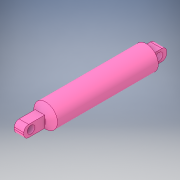
# Autodesk Inventor part: MockShock2
Saved by Autodesk Inventor 2018.2 (Build 222227000, 227)
## iProperties
Created: 2018-03-24
Part Number: MockShock2
Material: Generic
Document SubType Name: Modeling
Designer: MIABo
Density: 1 g/cm^3
Appearance: Default
Author: MIABo
Autodesk Inventor part; units mm, degrees
ref_plane "YZ Plane" through (0, 0, 0) normal (1, 0, 0) x (0, 1, 0)
ref_plane "XZ Plane" through (0, 0, 0) normal (0, 1, 0) x (-1, 0, 0)
ref_plane "XY Plane" through (0, 0, 0) normal (0, 0, 1) x (1, 0, 0)
sketch "Sketch1" plane through (0, 0, 0) normal (0, 0, 1) x (1, 0, 0)
  circle A0 centre (0, 0) radius 7.874
  dimension "d0" = 15.748
  constraints: 1 centre point, 1 coincident
  measures "d0" diameter of A0
extrude "Extrusion1" add sketch "Sketch1" along normal blind 67.31
ref_plane "Work Plane1" through (0, 0, 71.12) normal (0, 0, 1) x (1, 0, 0)
sketch "Sketch3" plane through (0, 0, 71.12) normal (0, 0, 1) x (1, 0, 0)
  circle A0 centre (0, 0) radius 3.81
  dimension "d4" = 7.62
  constraints: 1 centre point, 1 coincident
  measures "d4" diameter of A0
loft "Loft1" add profiles "Sketch3" section 1 edges at (-7.874, 0, 67.31)
ref_plane "Work Plane5" through (0, 0, 85.09) normal (0, 0, 1) x (1, 0, 0)
ref_plane "Work Plane8" through (4.445, 0, 85.09) normal (1, 0, 0) x (0, 1, 0)
sketch "Sketch6" plane through (4.445, 0, 85.09) normal (1, 0, 0) x (0, 1, 0)
  line L0 (4.445, 0) -> (-4.445, 0) projected
  point P0 (0, -85.09)
  point P1 (0, -4.826)
  dimension "d23" = 4.826
  measures "d23" distance from line of L0 point (0, -4.826)
ref_plane "Work Plane6" through (4.445, 0, 85.09) normal (1, 0, 0) x (0, 1, 0)
sketch "Sketch8" plane through (4.445, 0, 85.09) normal (1, 0, 0) x (0, 1, 0)
  line L0 (-5.08, -94.742) -> (5.08, -94.742) projected
  point P0 (0, -85.09)
  point P1 (0, -89.662)
  dimension "d31" = 5.08
  measures "d31" distance from line of L0 point (0, -89.662)
sketch "Sketch9" plane through (0, 0, 0) normal (0, 0, -1) x (-1, 0, 0)
  line L0 (-3.81, 3.81) -> (3.81, 3.81)
  line L1 (3.81, 3.81) -> (3.81, -3.81)
  line L2 (3.81, -3.81) -> (-3.81, -3.81)
  line L3 (-3.81, -3.81) -> (-3.81, 3.81)
  line L4 (-3.81, 3.81) -> (3.81, -3.81) construction
  line L5 (3.81, 3.81) -> (-3.81, -3.81) construction
  point P0 (0, 0)
  dimension "d39" = 7.62
  dimension "d40" = 7.62
  constraints: 12 end point, 2 midpoint, 2 parallel, 1 horizontal, 1 perpendicular
  measures "d39" distance of L0.end L1.end
  measures "d40" distance of L0.start L0.end
extrude "Extrusion6" add sketch "Sketch9" along normal blind 9.652
hole "Hole3" at (4.445, 0, -4.572) direction (-1, 0, 0) diameter 5.08 end through all both
sketch "Sketch10" plane through (0, 0, 71.12) normal (0, 0, 1) x (1, 0, 0)
  line L0 (3.175, 3.81) -> (-3.175, 3.81)
  line L1 (-3.175, 3.81) -> (-3.175, -3.81)
  line L2 (-3.175, -3.81) -> (3.175, -3.81)
  line L3 (3.175, -3.81) -> (3.175, 3.81)
  line L4 (3.175, 3.81) -> (-3.175, -3.81) construction
  line L5 (-3.175, 3.81) -> (3.175, -3.81) construction
  point P0 (0, 0)
  point P1 (0, 0)
  dimension "d50" = 6.35
  dimension "d51" = 7.62
  constraints: 12 end point, 2 midpoint, 2 parallel, 1 horizontal, 1 perpendicular
  measures "d50" distance of L2.end L1.end
  measures "d51" distance of L1.end L0.end
extrude "Extrusion7" add sketch "Sketch10" along normal blind 13.97
hole "Hole4" at (4.445, 0, 80.264) direction (-1, 0, 0) diameter 5.08 end through all
fillet "Fillet1" radius 3.175 2 edges at (0, 3.81, 85.09) (0, -3.81, 85.09)
fillet "Fillet2" radius 3.175 2 edges at (0, 3.81, -9.652) (0, -3.81, -9.652)
body "Solid1"
